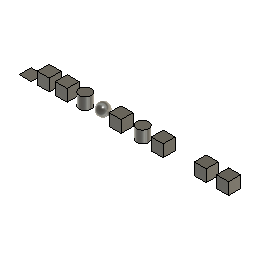
Plane 생성 교육용 v2 (Autodesk Fusion 360 design; units mm, degrees)
Autodesk Fusion 360 part; units mm, degrees
sketch "Sketch1" plane through (0, 0, 0) normal (0, 0, 1) x (1, 0, 0)
  line L0 (-80, 10) -> (-60, 10)
  line L1 (-60, 10) -> (-60, -10)
  line L2 (-60, -10) -> (-80, -10)
  line L3 (-80, -10) -> (-80, 10)
  constraint horizontal L0
  constraint vertical L1
  constraint horizontal L2
  constraint vertical L3
surface "SurfacePatch1" add patch profiles "Sketch1" section 1 makes body 1
box "BoxPrimitive1" add length 20 width 20 height 20 placed x (0, -1, 0) y (1, 0, 0) z (0, 0, 1) at (-50, 10, 0) separate body makes body 2
cylinder "CylinderPrimitive1" add diameter 20 height 20 placed x (1, 0, 0) y (0, 1, 0) z (0, 0, 1) at (-10, 0, 0) separate body makes body 3
sphere "SpherePrimitive1" add diameter 20 placed x (1, 0, 0) y (0, 1, 0) z (0, 0, 1) at (20, 0, 0) separate body makes body 4
move_body "Move1" bodies 4 to x (1, 0, 0) y (0, 1, 0) z (0, 0, 1) at (0, 0, 10)
move_body "Move2" bodies 1 2 to x (1, 0, 0) y (0, 1, 0) z (0, 0, 1) at (-30, 0, 0)
copy_body "CopyPasteBodies1" bodies 2 makes body 5
move_body "Move3" bodies 5 to x (1, 0, 0) y (0, 1, 0) z (0, 0, 1) at (30, 0, 0)
ref_plane "WorkPlane2" through (-100, 0, 10) normal (0, 0, 1) x (1, 0, 0)
ref_plane "WorkPlane3" through (-100, 0, 20) normal (0, 0, 1) x (1, 0, 0)
ref_plane "WorkPlane4" through (-70, 10, 20) normal (0, 0.766044, 0.642788) x (-1, 0, 0)
ref_plane "WorkPlane5" through (-70, -10, 20) normal (0, -0.766044, 0.642788) x (1, 0, 0)
ref_plane "WorkPlane6" through (-20, 0, 10.4887) normal (-1, 0, 0) x (0, 1, 0)
ref_plane "WorkPlane7" through (0, 0, 13.6981) normal (1, 0, 0) x (0, -1, 0)
ref_plane "WorkPlane8" through (-10, -10, 13.7783) normal (0, -1, 0) x (-1, 0, 0)
ref_plane "WorkPlane9" through (-10, 10, 10.6363) normal (0, 1, 0) x (1, 0, 0)
ref_plane "WorkPlane10" through (-40, 0, 10) normal (-1, 0, 0) x (0, 0, -1)
ref_plane "WorkPlane11" through (-40, 0, 10) normal (0, -1, 0) x (0, 0, -1)
copy_body "CopyPasteBodies2" bodies 5 makes body 6
move_body "Move4" bodies 6 to x (1, 0, 0) y (0, 1, 0) z (0, 0, 1) at (90, 0, 0)
ref_plane "WorkPlane12" through (60, 10, 20) normal (0, 0.707107, -0.707107) x (-1, 0, 0)
ref_plane "WorkPlane13" through (40, 10, 20) normal (0.707107, 0, 0.707107) x (0, 1, 0)
copy_body "CopyPasteBodies3" bodies 3 makes body 7
move_body "Move5" bodies 7 to x (1, 0, 0) y (0, 1, 0) z (0, 0, 1) at (96.0187, 0, 0)
copy_body "CopyPasteBodies4" bodies 6 makes body 8
move_body "Move6" bodies 8 to x (1, 0, 0) y (0, 1, 0) z (0, 0, 1) at (70.2088, 0, 0)
ref_plane "WorkPlane14" through (156.7146, 0, 28.729) normal (0, 0, 1) x (0, -1, 0)
ref_plane "WorkPlane15" through (156.7146, -19.612, 10) normal (0, -1, 0) x (0, 0, -1)
copy_body "CopyPasteBodies6" bodies 8 makes body 9
move_body "Move8" bodies 9 to x (1, 0, 0) y (0, 1, 0) z (0, 0, 1) at (71.9223, 0, 0)
copy_body "CopyPasteBodies7" bodies 9 makes body 10
move_body "Move9" bodies 10 to x (1, 0, 0) y (0, 1, 0) z (0, 0, 1) at (37.2621, 0, 0)
